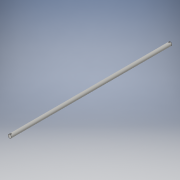
# Autodesk Inventor part: Straw Hyp
Saved by Autodesk Inventor 2016 (Build 200138000, 138)
## iProperties
Created: 2017-04-28
Part Number: Straw Hyp
Material: Generic
Document SubType Name: Modeling
Designer: wtse3759
Density: 1 g/cm^3
Appearance: Default
Author: wtse3759
Autodesk Inventor part; units mm, degrees
ref_plane "YZ Plane" through (0, 0, 0) normal (1, 0, 0) x (0, 1, 0)
ref_plane "XZ Plane" through (0, 0, 0) normal (0, 1, 0) x (-1, 0, 0)
ref_plane "XY Plane" through (0, 0, 0) normal (0, 0, 1) x (1, 0, 0)
sketch "Sketch1" plane through (0, 0, 0) normal (0, 0, 1) x (1, 0, 0)
  circle A0 centre (0, 0) radius 3.175
  dimension "d0" = 6.35
  constraints: 1 centre point, 1 coincident
  measures "d0" diameter of A0
extrude "Extrusion1" add sketch "Sketch1" along normal blind 287.3682
sketch "Sketch2" plane through (0, 0, 0) normal (0, 1, 0) x (-1, 0, 0)
  line L0 (0, 0) -> (0, 1.524)
  circle A0 centre (0, 1.524) radius 1.27
  line L1 (3.175, 287.3682) -> (-3.175, 287.3682) projected
  line L2 (0, 287.3682) -> (0, 285.8442)
  circle A1 centre (0, 285.8442) radius 1.27
  dimension "d3" = 1.524
  dimension "d4" = 2.54
  dimension "d5" = 1.524
  dimension "d6" = 2.54
  constraints: 4 end point, 2 centre point, 2 coincident, 2 vertical, 1 midpoint
  measures "d3" distance of L0.start L0.end
  measures "d4" diameter of A0
  measures "d5" distance of L2.start L2.end
  measures "d6" diameter of A1
extrude "Extrusion2" cut sketch "Sketch2" along normal mid plane 7.62
body "Solid1"
